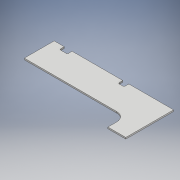
# Autodesk Inventor part: TableOlya
Saved by Autodesk Inventor 2018 (Build 220112000, 112)
## iProperties
Created: 2018-08-12
Part Number: TableOlya
Material: Generic
Document SubType Name: Modeling
Designer: Toshiba
Density: 1 g/cm^3
Appearance: Default
Author: Toshiba
Autodesk Inventor part; units mm, degrees
ref_plane "YZ Plane" through (0, 0, 0) normal (1, 0, 0) x (0, 1, 0)
ref_plane "XZ Plane" through (0, 0, 0) normal (0, 1, 0) x (-1, 0, 0)
ref_plane "XY Plane" through (0, 0, 0) normal (0, 0, 1) x (1, 0, 0)
sketch "Sketch1" plane through (0, 0, 0) normal (0, 0, 1) x (1, 0, 0)
  line L0 (1000, 500) -> (1000, 0)
  line L1 (-1000, 0) -> (-1000, 500)
  line L2 (700, -300) -> (1000, -300)
  line L3 (1000, -300) -> (1000, 0)
  line L4 (-1000, 0) -> (550, 0)
  line L5 (700, -300) -> (700, -150)
  arc A0 (700, -150) -> (550, 0) centre (550, -150) ccw
  line L6 (250, 500) -> (1000, 500)
  line L7 (150, 500) -> (150, 440)
  line L8 (250, 440) -> (250, 500)
  line L9 (-1000, 500) -> (-830, 500)
  line L10 (-830, 500) -> (-830, 440)
  line L11 (-810, 420) -> (-720, 420)
  line L12 (-700, 440) -> (-700, 500)
  line L13 (-700, 500) -> (150, 500)
  line L14 (170, 420) -> (230, 420)
  arc A1 (-720, 420) -> (-700, 440) centre (-720, 440) ccw
  arc A2 (-830, 440) -> (-810, 420) centre (-810, 440) ccw
  arc A3 (150, 440) -> (170, 420) centre (170, 440) ccw
  arc A4 (230, 420) -> (250, 440) centre (230, 440) ccw
  point P0 (0, 0)
  point P1 (150, 420)
  point P2 (250, 420)
  point P3 (-830, 420)
  point P4 (-700, 420)
  dimension "d2" = 2000
  dimension "d3" = 500
  dimension "d4" = 300
  dimension "d5" = 300
  dimension "d6" = 150
  dimension "d7" = 1550
  dimension "d8" = 150
  dimension "d11" = 80
  dimension "d12" = 100
  dimension "d13" = 170
  dimension "d14" = 80
  dimension "d15" = 130
  dimension "d16" = 850
  dimension "d18" = 20
  dimension "d19" = 20
  dimension "d20" = 20
  dimension "d21" = 20
  constraints: 30 end point, 10 point on circle, 9 tangent, 8 point on line, 5 centre point, 5 horizontal, 3 perpendicular, 3 vertical, 1 parallel
  measures "d2" distance of L0.end L1.start
  measures "d3" distance of L0.start L0.end
  measures "d4" distance of L2.start L2.end
  measures "d5" distance of L2.end L0.end
  measures "d6" distance of L5.end L2.start
  measures "d7" distance of L1.start L4.end
  measures "d8" radius of A0
  measures "d11" distance of L7.start point (150, 420)
  measures "d12" distance of point (150, 420) point (250, 420)
  measures "d13" distance of L1.end L9.end
  measures "d14" distance of L9.end point (-830, 420)
  measures "d15" distance of point (-830, 420) point (-700, 420)
  measures "d16" distance of L12.end L7.start
  measures "d18" radius of A1
  measures "d19" radius of A2
  measures "d20" radius of A3
  measures "d21" radius of A4
extrude "Extrusion1" add sketch "Sketch1" along normal blind 25
body "Solid1"
